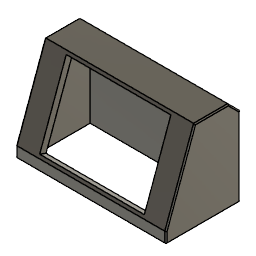
lcd holder_v1 (Autodesk Fusion 360 design; units mm, degrees)
Autodesk Fusion 360 part; units mm, degrees
sketch "Sketch1" plane through (0, 0, 0) normal (1, 0, 0) x (0, 1, 0)
  line L0 (0, 0) -> (0, 5)
  line L1 (0, 5) -> (12.6547, 39.7686)
  line L2 (0, 5) -> (37, 5) construction
  line L3 (12.6547, 39.7686) -> (32.6547, 39.7686)
  line L4 (32.6547, 39.7686) -> (32.6547, 0)
  line L5 (32.6547, 0) -> (0, 0)
  dimension "d1" = 70
  dimension "d2" = 37
  dimension "d3" = 20
  constraint coincident L0.start L5.end
  constraint vertical L0
  constraint horizontal L2
  constraint horizontal L3
  constraint perpendicular L2 L4
  constraint perpendicular L0 L5
  measures "d1" angle of L1 L2
  measures "d2" distance of L0.end L1.end
  measures "d3" distance of L1.end L3.end
extrude "Extrude1" add sketch "Sketch1" along normal mid plane 66
shell "Shell1" thickness 3 removed faces 1 at (11, 10.8849, 0)
chamfer "Chamfer1" distance 5 angle 45 1 edges at (0, 32.6547, 39.7686)
chamfer "Chamfer1" distance 0.5 angle 45 6 edges at (33, 22.6547, 39.7686) (-33, 22.6547, 39.7686) (0, 32.6547, 0) (33, 16.3274, 0) (0, 0, 0) (-33, 16.3274, 0)
fillet "Fillet1" radius 0.5 8 edges at (-33, 6.2364, 22.1343) (33, 6.2364, 22.1343) (-33, 32.6547, 17.6343) (33, 32.6547, 17.6343) (33, 30.4047, 37.0186) (-33, 30.4047, 37.0186) (-33, 0, 2.75) (33, 0, 2.75)
sketch "Sketch2" plane through (0, -1.607, 0.5849) normal (0, -0.939693, 0.34202) x (1, 0, 0)
  line L0 (32.5, 4.6985) -> (32.5, 41.6985)
  line L1 (32.5, 41.6985) -> (-32.5, 41.6985)
  line L2 (-32.5, 41.6985) -> (-32.5, 4.6985)
  line L3 (-32.5, 4.6985) -> (32.5, 4.6985)
  line L4 (-32.5, 41.6985) -> (32.5, 4.6985) construction
  line L5 (32.5, 41.6985) -> (-32.5, 4.6985) construction
  line L6 (23, 40.2985) -> (-23, 40.2985)
  line L7 (-23, 40.2985) -> (-23, 6.0985)
  line L8 (-23, 6.0985) -> (23, 6.0985)
  line L9 (23, 6.0985) -> (23, 40.2985)
  line L10 (23, 40.2985) -> (-23, 6.0985) construction
  line L11 (-23, 40.2985) -> (23, 6.0985) construction
  point P0 (0, 23.1985)
  dimension "d13" = 46
  dimension "d14" = 34.2
  constraint coincident L1.end L2.start
  constraint coincident L0.start L3.end
  constraint coincident L0.end L1.start
  constraint coincident L2.end L3.start
  constraint horizontal L6
  constraint perpendicular L6 L7
  constraint parallel L6 L8
  constraint parallel L7 L9
  constraint coincident L10 P0
  constraint coincident L11 P0
  constraint midpoint L4 P0
  measures "d13" distance of L7.end L8.end
  measures "d14" distance of L6.end L7.end
extrude "Extrude2" cut sketch "Sketch2" against normal blind 6 contours L6 L7 L8 L9
